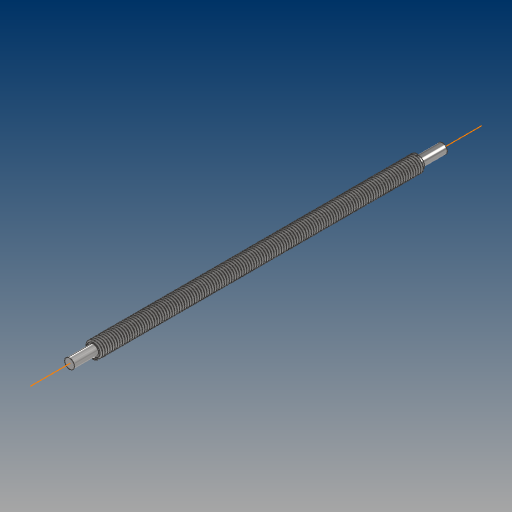
# Autodesk Inventor part: Vit_me_300x12
Saved by Autodesk Inventor 2021 (Build 250183000, 183)
## iProperties
Created: 2024-04-07
Part Number: Vit_me_300x12
Material: Stainless Steel, Austenitic
Document SubType Name: Modeling
Designer: Admin
Density: 8 g/cm^3
Appearance: Semi-Polished
Mass: 214.468 g
Surface Area: 171.453 cm^2
Volume: 26.8085 cm^3
Author: Admin
Autodesk Inventor part; units mm, degrees
ref_plane "YZ Plane" through (0, 0, 0) normal (1, 0, 0) x (0, 1, 0)
ref_plane "XZ Plane" through (0, 0, 0) normal (0, 1, 0) x (-1, 0, 0)
ref_plane "XY Plane" through (0, 0, 0) normal (0, 0, 1) x (1, 0, 0)
sketch "Sketch1" plane through (0, 0, 0) normal (1, 0, 0) x (0, 1, 0)
  line L0 (0, 181.6581) -> (0, -118.3419)
  line L1 (0, 181.6581) -> (4, 181.6581)
  line L2 (4, 181.6581) -> (4, 162.2581)
  line L3 (4, 162.2581) -> (5, 162.2581)
  line L4 (5, 162.2581) -> (5, -98.9419)
  line L5 (5, -98.9419) -> (4, -98.9419)
  line L6 (4, -98.9419) -> (4, -118.3419)
  line L7 (4, -118.3419) -> (0, -118.3419)
  point P0 (0, 0)
  dimension "d0" = 4
  dimension "d1" = 19.4
  dimension "d2" = 300
  dimension "d3" = 5
  constraints: 16 end point, 5 perpendicular, 2 point on line, 1 collinear, 1 horizontal, 1 vertical
  measures "d0" distance of L6.end L0.end
  measures "d1" distance between parallel lines of L7 L5
  measures "d2" distance between parallel lines of L7 L1
  measures "d3" distance between parallel lines of L0 L4
revolve "Revolution1" add sketch "Sketch1" angle 360 about axis through (0, 0, 181.6581) along (0, 0, -1)
sketch "Sketch2" plane through (0, 0, 0) normal (1, 0, 0) x (0, 1, 0)
  line L0 (-5, 162.2581) -> (5, 162.2581) projected
  line L1 (-5, -98.9419) -> (5, -98.9419) projected
  line L2 (5, 162.2581) -> (5, -98.9419) projected
  line L3 (-5, 162.2581) -> (-5, -98.9419) projected
  line L4 (5, -97.4419) -> (6.299, -98.1919)
  line L5 (-5, -98.9419) -> (5, -98.9419) projected
  line L6 (6.299, -98.1919) -> (5, -98.9419)
  point P0 (0, 0)
  dimension "d5" = 261.2
  dimension "d6" = 60
  dimension "d7" = 1.5
  constraints: 4 end point, 1 equal length, 1 point on line
  measures "d5" distance of L2.start L2.end
  measures "d6" angle of L6 L4
  measures "d7" distance of L4.start L1.end
coil "Coil1" sketch "Sketch2" operation add axis through (0, 0, -10) along (0, 0, 1) pitch 2 turns 130.6 hand right contours L4 L6 L2
equation "\"d9\" = d5"
body "Solid1"
